Autodesk Inventor part; units mm, degrees
(part 4 of 4)
  arc A543 (17.8769, 14.9832) -> (17.4024, 14.8775) centre (19.2881, 7.5282) ccw projected
  arc A544 (17.4024, 14.8775) -> (17.024, 14.7679) centre (18.9945, 8.6707) ccw projected
  arc A545 (17.024, 14.7679) -> (16.7289, 14.6628) centre (18.6448, 9.7513) ccw projected
  arc A546 (16.7289, 14.6628) -> (16.506, 14.9696) centre (0.9435, 3.4284) ccw projected
  arc A547 (16.506, 14.9696) -> (16.6971, 15.2177) centre (12.4269, 18.3094) ccw projected
  arc A548 (16.6971, 15.2177) -> (16.9183, 15.5438) centre (11.5073, 18.976) ccw projected
  arc A549 (16.9183, 15.5438) -> (17.1654, 15.9624) centre (10.5114, 19.6082) ccw projected
  arc A550 (17.1654, 15.9624) -> (16.9181, 16.2761) centre (0.9435, 3.4284) ccw projected
  arc A551 (16.9181, 16.2761) -> (16.4534, 16.1335) centre (18.9098, 8.9549) ccw projected
  arc A552 (16.4534, 16.1335) -> (16.0847, 15.9946) centre (18.5276, 10.0708) ccw projected
  arc A553 (16.0847, 15.9946) -> (15.7988, 15.8667) centre (18.0941, 11.1207) ccw projected
  arc A554 (15.7988, 15.8667) -> (15.5525, 16.1551) centre (0.9435, 3.4284) ccw projected
  arc A555 (15.5525, 16.1551) -> (15.7236, 16.4174) centre (11.224, 19.1645) ccw projected
  arc A556 (15.7236, 16.4174) -> (15.9185, 16.7598) centre (10.2549, 19.7569) ccw projected
  arc A557 (15.9185, 16.7598) -> (16.132, 17.1965) centre (9.2125, 20.309) ccw projected
  arc A558 (16.132, 17.1965) -> (15.8608, 17.4899) centre (0.9435, 3.4284) ccw projected
  arc A559 (15.8608, 17.4899) -> (15.4087, 17.3113) centre (18.4209, 10.3475) ccw projected
  arc A560 (15.4087, 17.3113) -> (15.0521, 17.1438) centre (17.9522, 11.43) ccw projected
  arc A561 (15.0521, 17.1438) -> (14.7772, 16.9939) centre (17.4377, 12.4426) ccw projected
  arc A562 (14.7772, 16.9939) -> (14.509, 17.2621) centre (0.9435, 3.4284) ccw projected
  arc A563 (14.509, 17.2621) -> (14.6589, 17.537) centre (9.9577, 19.9226) ccw projected
  arc A564 (14.6589, 17.537) -> (14.8264, 17.8936) centre (8.9451, 20.4371) ccw projected
  arc A565 (14.8264, 17.8936) -> (15.005, 18.3458) centre (7.8625, 20.9058) ccw projected
  arc A566 (15.005, 18.3458) -> (14.7116, 18.6169) centre (0.9435, 3.4284) ccw projected
  arc A567 (14.7116, 18.6169) -> (14.2749, 18.4034) centre (17.8241, 11.6974) ccw projected
  arc A568 (14.2749, 18.4034) -> (13.9325, 18.2085) centre (17.272, 12.7398) ccw projected
  arc A569 (13.9325, 18.2085) -> (13.6702, 18.0374) centre (16.6796, 13.7089) ccw projected
  arc A570 (13.6702, 18.0374) -> (13.3818, 18.2837) centre (0.9435, 3.4284) ccw projected
  arc A571 (13.3818, 18.2837) -> (13.5097, 18.5696) centre (8.6357, 20.579) ccw projected
  arc A572 (13.5097, 18.5696) -> (13.6486, 18.9383) centre (7.5859, 21.0125) ccw projected
  arc A573 (13.6486, 18.9383) -> (13.7912, 19.403) centre (6.47, 21.3947) ccw projected
  arc A574 (13.7912, 19.403) -> (13.4775, 19.6503) centre (0.9435, 3.4284) ccw projected
  arc A575 (13.4775, 19.6503) -> (13.0589, 19.4032) centre (17.1233, 12.9963) ccw projected
  arc A576 (13.0589, 19.4032) -> (12.7328, 19.182) centre (16.4911, 13.9922) ccw projected
  arc A577 (12.7328, 19.182) -> (12.4847, 18.9909) centre (15.8245, 14.9118) ccw projected
  arc A578 (12.4847, 18.9909) -> (12.1779, 19.2138) centre (0.9435, 3.4284) ccw projected
  arc A579 (12.1779, 19.2138) -> (12.283, 19.5089) centre (7.2664, 21.1297) ccw projected
  arc A580 (12.283, 19.5089) -> (12.3926, 19.8873) centre (6.1858, 21.4794) ccw projected
  arc A581 (12.3926, 19.8873) -> (12.4983, 20.3618) centre (5.0433, 21.773) ccw projected
  arc A582 (12.4983, 20.3618) -> (12.1661, 20.5837) centre (0.9435, 3.4284) ccw projected
  arc A583 (12.1661, 20.5837) -> (11.7682, 20.3045) centre (16.3227, 14.2363) ccw projected
  arc A584 (11.7682, 20.3045) -> (11.4605, 20.0585) centre (15.6143, 15.1795) ccw projected
  arc A585 (11.4605, 20.0585) -> (11.2281, 19.8485) centre (14.8777, 16.044) ccw projected
  arc A586 (11.2281, 19.8485) -> (10.9048, 20.0466) centre (0.9435, 3.4284) ccw projected
  arc A587 (10.9048, 20.0466) -> (10.9864, 20.349) centre (5.8581, 21.5712) ccw projected
  arc A588 (10.9864, 20.349) -> (11.0659, 20.7348) centre (4.7534, 21.8351) ccw projected
  arc A589 (11.0659, 20.7348) -> (11.1341, 21.2162) centre (3.5914, 22.0381) ccw projected
  arc A590 (11.1341, 21.2162) -> (10.7855, 21.4113) centre (0.9435, 3.4284) ccw projected
  arc A591 (10.7855, 21.4113) -> (10.4107, 21.1018) centre (15.4274, 15.4096) ccw projected
  arc A592 (10.4107, 21.1018) -> (10.1233, 20.8323) centre (14.6471, 16.2943) ccw projected
  arc A593 (10.1233, 20.8323) -> (9.9081, 20.6048) centre (13.8449, 17.0984) ccw projected
  arc A594 (9.9081, 20.6048) -> (9.5702, 20.7769) centre (0.9435, 3.4284) ccw projected
  arc A595 (9.5702, 20.7769) -> (9.6279, 21.0848) centre (4.4195, 21.9009) ccw projected
  arc A596 (9.6279, 21.0848) -> (9.6769, 21.4757) centre (3.2975, 22.0773) ccw projected
  arc A597 (9.6769, 21.4757) -> (9.707, 21.9609) centre (2.1231, 22.1885) ccw projected
  arc A598 (9.707, 21.9609) -> (9.3443, 22.1281) centre (0.9435, 3.4284) ccw projected
  arc A599 (9.3443, 22.1281) -> (8.9949, 21.7901) centre (14.4427, 16.5091) ccw projected
  arc A600 (8.9949, 21.7901) -> (8.7295, 21.4989) centre (13.5955, 17.3298) ccw projected
  arc A601 (8.7295, 21.4989) -> (8.5329, 21.2552) centre (12.7326, 18.0685) ccw projected
  arc A602 (8.5329, 21.2552) -> (8.1825, 21.4003) centre (0.9435, 3.4284) ccw projected
  arc A603 (8.1825, 21.4003) -> (8.2158, 21.7117) centre (2.9594, 22.1166) ccw projected
  arc A604 (8.2158, 21.7117) -> (8.234, 22.1053) centre (1.827, 22.2045) ccw projected
  arc A605 (8.234, 22.1053) -> (8.226, 22.5913) centre (0.6476, 22.2232) ccw projected
  arc A606 (8.226, 22.5913) -> (7.8512, 22.7296) centre (0.9435, 3.4284) ccw projected
  arc A607 (7.8512, 22.7296) -> (7.5294, 22.3652) centre (13.3748, 17.5279) ccw projected
  arc A608 (7.5294, 22.3652) -> (7.2877, 22.0541) centre (12.4658, 18.2796) ccw projected
  arc A609 (7.2877, 22.0541) -> (7.1108, 21.7957) centre (11.5476, 18.9483) ccw projected
  arc A610 (7.1108, 21.7957) -> (6.7501, 21.9129) centre (0.9435, 3.4284) ccw projected
  arc A611 (6.7501, 21.9129) -> (6.7589, 22.2259) centre (1.487, 22.2172) ccw projected
  arc A612 (6.7589, 22.2259) -> (6.7462, 22.6197) centre (0.3512, 22.2159) ccw projected
  arc A613 (6.7462, 22.6197) -> (6.7, 23.1036) centre (-0.8261, 22.142) ccw projected
  arc A614 (6.7, 23.1036) -> (6.3156, 23.212) centre (0.9435, 3.4284) ccw projected
  arc A615 (6.3156, 23.212) -> (6.0234, 22.8235) centre (12.2302, 18.4597) ccw projected
  arc A616 (6.0234, 22.8235) -> (5.8068, 22.4944) centre (11.265, 19.1379) ccw projected
  arc A617 (5.8068, 22.4944) -> (5.6507, 22.2229) centre (10.2973, 19.7324) ccw projected
  arc A618 (5.6507, 22.2229) -> (5.2819, 22.3115) centre (0.9435, 3.4284) ccw projected
  arc A619 (5.2819, 22.3115) -> (5.2661, 22.6242) centre (0.0111, 22.2019) ccw projected
  arc A620 (5.2661, 22.6242) -> (5.2225, 23.0158) centre (-1.121, 22.1115) ccw projected
  arc A621 (5.2225, 23.0158) -> (5.1386, 23.4946) centre (-2.2889, 21.9455) ccw projected
  arc A622 (5.1386, 23.4946) -> (4.7468, 23.5725) centre (0.9435, 3.4284) ccw projected
  arc A623 (4.7468, 23.5725) -> (4.486, 23.1623) centre (11.0161, 19.299) ccw projected
  arc A624 (4.486, 23.1623) -> (4.2959, 22.8172) centre (10.0007, 19.8993) ccw projected
  arc A625 (4.2959, 22.8172) -> (4.1616, 22.5343) centre (8.9892, 20.4161) ccw projected
  arc A626 (4.1616, 22.5343) -> (3.787, 22.5936) centre (0.9435, 3.4284) ccw projected
  arc A627 (3.787, 22.5936) -> (3.7467, 22.9042) centre (-1.4589, 22.0709) ccw projected
  arc A628 (3.7467, 22.9042) -> (3.6725, 23.2911) centre (-2.5805, 21.8919) ccw projected
  arc A629 (3.6725, 23.2911) -> (3.5513, 23.7619) centre (-3.7318, 21.6348) ccw projected
  arc A630 (3.5513, 23.7619) -> (3.1546, 23.8088) centre (0.9435, 3.4284) ccw projected
  arc A631 (3.1546, 23.8088) -> (2.9268, 23.3794) centre (9.7398, 20.0403) ccw projected
  arc A632 (2.9268, 23.3794) -> (2.7643, 23.0205) centre (8.6805, 20.5591) ccw projected
  arc A633 (2.7643, 23.0205) -> (2.6526, 22.7279) centre (7.6316, 20.995) ccw projected
  arc A634 (2.6526, 22.7279) -> (2.2746, 22.7577) centre (0.9435, 3.4284) ccw projected
  arc A635 (2.2746, 22.7577) -> (2.21, 23.0641) centre (-2.9142, 21.8249) ccw projected
  arc A636 (2.21, 23.0641) -> (2.1057, 23.444) centre (-4.0183, 21.5585) ccw projected
  arc A637 (2.1057, 23.444) -> (1.9479, 23.9038) centre (-5.1458, 21.2118) ccw projected
  arc A638 (1.9479, 23.9038) -> (1.5487, 23.9195) centre (0.9435, 3.4284) ccw projected
  arc A639 (1.5487, 23.9195) -> (1.3553, 23.4735) centre (8.4094, 20.6793) ccw projected
  arc A640 (1.3553, 23.4735) -> (1.2215, 23.1029) centre (7.3125, 21.1133) ccw projected
  circle A641 centre (0.9435, 3.4284) radius 20.5
  circle A642 centre (0.9435, 3.4284) radius 18.25
  circle A643 centre (0.9435, 3.4284) radius 5
  point P0 (0, 0)
  dimension "d5" = 41
  dimension "d6" = 2.25
  dimension "d7" = 10
  constraints: 3 centre point, 2 coincident
  measures "d5" diameter of A641
  measures "d6" radial gap between concentric circles of A641 A642
  measures "d7" diameter of A643
extrude "押し出し3" cut sketch "スケッチ3" against normal blind 0.75 contours A0 | A642
sketch "スケッチ4" plane through (0, 0, 0) normal (0, 0, -1) x (-1, 0, 0)
  circle A0 centre (-0.9435, 3.4284) radius 8 projected
  circle A1 centre (-0.9435, 3.4284) radius 18.25
  circle A2 centre (-0.9435, 3.4284) radius 5
  point P0 (0, 0)
  dimension "d10" = 36.5
  dimension "d11" = 10
  constraints: 2 centre point, 2 coincident
  measures "d10" diameter of A1
  measures "d11" diameter of A2
extrude "押し出し4" cut sketch "スケッチ4" against normal blind 0.75 contours A0 | A1
sketch "スケッチ5" plane through (0.9435, 3.4284, 0.75) normal (0, 0, -1) x (-1, 0, 0)
  circle A0 centre (-14, 0) radius 1.25
  circle A1 centre (0, 14) radius 1.25
  circle A2 centre (14, 0) radius 1.25
  circle A3 centre (0, -14) radius 1.25
  circle A4 centre (0, 0) radius 17.5 projected
  arc A5 (-1.7867, -11.2539) -> (-1.3867, -10.4941) centre (-4.7153, -9.2268) ccw projected
  arc A6 (-1.3867, -10.4941) -> (-1.3184, -10.2522) centre (-2.5769, -10.0277) ccw projected
  line L0 (-1.3184, -10.2522) -> (-1.0841, -8.4306) projected
  arc A7 (-1.0841, -8.4306) -> (1.0841, -8.4306) centre (0, 0) ccw projected
  line L1 (1.0841, -8.4306) -> (1.3184, -10.2522) projected
  arc A8 (1.3184, -10.2522) -> (1.3867, -10.4941) centre (2.5769, -10.0277) ccw projected
  arc A9 (1.3867, -10.4941) -> (1.7867, -11.2539) centre (4.7153, -9.2268) ccw projected
  arc A10 (1.7867, -11.2539) -> (3.0777, -12.6304) centre (7.0036, -7.6547) ccw projected
  arc A11 (3.0777, -12.6304) -> (4.2394, -12.2893) centre (0, 0) ccw projected
  arc A12 (4.2394, -12.2893) -> (4.5813, -10.4334) centre (-1.7533, -10.226) ccw projected
  arc A13 (4.5813, -10.4334) -> (4.507, -9.5779) centre (1.0216, -10.3114) ccw projected
  arc A14 (4.507, -9.5779) -> (4.4336, -9.3375) centre (3.2536, -9.829) ccw projected
  line L2 (4.4336, -9.3375) -> (3.6459, -7.6784) projected
  arc A15 (3.6459, -7.6784) -> (5.47, -6.5061) centre (0, 0) ccw projected
  line L3 (5.47, -6.5061) -> (6.6519, -7.9119) projected
  arc A16 (6.6519, -7.9119) -> (6.8401, -8.0785) centre (7.5892, -7.0426) ccw projected
  arc A17 (6.8401, -8.0785) -> (7.5874, -8.5014) centre (8.9551, -5.2128) ccw projected
  arc A18 (7.5874, -8.5014) -> (9.4177, -8.9614) centre (10.0302, -2.6531) ccw projected
  arc A19 (9.4177, -8.9614) -> (10.2105, -8.0465) centre (0, 0) ccw projected
  arc A20 (10.2105, -8.0465) -> (9.4947, -6.3003) centre (4.0536, -9.5506) ccw projected
  arc A21 (9.4947, -6.3003) -> (8.9697, -5.6208) centre (6.4342, -8.1221) ccw projected
  arc A22 (8.9697, -5.6208) -> (8.778, -5.4582) centre (8.051, -6.5096) ccw projected
  line L4 (8.778, -5.4582) -> (7.2184, -4.4884) projected
  arc A23 (7.2184, -4.4884) -> (8.1191, -2.516) centre (0, 0) ccw projected
  line L5 (8.1191, -2.516) -> (9.8734, -3.0597) projected
  arc A24 (9.8734, -3.0597) -> (10.1218, -3.0981) centre (10.192, -1.8216) ccw projected
  arc A25 (10.1218, -3.0981) -> (10.9792, -3.0498) centre (10.3518, 0.4562) ccw projected
  arc A26 (10.9792, -3.0498) -> (12.7676, -2.4473) centre (9.8724, 3.1908) ccw projected
  arc A27 (12.7676, -2.4473) -> (12.9399, -1.2489) centre (0, 0) ccw projected
  arc A28 (12.9399, -1.2489) -> (11.3937, -0.1669) centre (8.5735, -5.8429) ccw projected
  arc A29 (11.3937, -0.1669) -> (10.5846, 0.1209) centre (9.8039, -3.3542) ccw projected
  arc A30 (10.5846, 0.1209) -> (10.3355, 0.1541) centre (10.2923, -1.1236) ccw projected
  line L6 (10.3355, 0.1541) -> (8.4991, 0.1267) projected
  arc A31 (8.4991, 0.1267) -> (8.1905, 2.2729) centre (0, 0) ccw projected
  line L7 (8.1905, 2.2729) -> (9.9602, 2.764) projected
  arc A32 (9.9602, 2.764) -> (10.1899, 2.866) centre (9.5589, 3.9777) ccw projected
  arc A33 (10.1899, 2.866) -> (10.8851, 3.3701) centre (8.4618, 5.9804) ccw projected
  arc A34 (10.8851, 3.3701) -> (12.0639, 4.8439) centre (6.5801, 8.0217) ccw projected
  arc A35 (12.0639, 4.8439) -> (11.5609, 5.9452) centre (0, 0) ccw projected
  arc A36 (11.5609, 5.9452) -> (9.6752, 6.0194) centre (10.3714, -0.2802) ccw projected
  arc A37 (9.6752, 6.0194) -> (8.839, 5.8242) centre (10.061, 2.4787) ccw projected
  arc A38 (8.839, 5.8242) -> (8.6115, 5.7174) centre (9.2659, 4.6193) ccw projected
  line L8 (8.6115, 5.7174) -> (7.0814, 4.7015) projected
  arc A39 (7.0814, 4.7015) -> (5.6614, 6.3402) centre (0, 0) ccw projected
  line L9 (5.6614, 6.3402) -> (6.8847, 7.7101) projected
  arc A40 (6.8847, 7.7101) -> (7.0228, 7.9201) centre (5.8909, 8.5142) ccw projected
  arc A41 (7.0228, 7.9201) -> (7.3351, 8.7201) centre (3.8853, 9.6058) ccw projected
  arc A42 (7.3351, 8.7201) -> (7.53, 10.5972) centre (1.1987, 10.3057) ccw projected
  arc A43 (7.53, 10.5972) -> (6.5115, 11.2517) centre (0, 0) ccw projected
  arc A44 (6.5115, 11.2517) -> (4.885, 10.2947) centre (8.8765, 5.3715) ccw projected
  arc A45 (4.885, 10.2947) -> (4.287, 9.6783) centre (7.1238, 7.5246) ccw projected
  arc A46 (4.287, 9.6783) -> (4.1534, 9.4655) centre (5.2976, 8.8955) ccw projected
  line L10 (4.1534, 9.4655) -> (3.4154, 7.7836) projected
  arc A47 (3.4154, 7.7836) -> (1.3349, 8.3945) centre (0, 0) ccw projected
  line L11 (1.3349, 8.3945) -> (1.6234, 10.2083) projected
  arc A48 (1.6234, 10.2083) -> (1.626, 10.4597) centre (0.3526, 10.3475) ccw projected
  arc A49 (1.626, 10.4597) -> (1.4563, 11.3015) centre (-1.9248, 10.1815) ccw projected
  arc A50 (1.4563, 11.3015) -> (0.6053, 12.9859) centre (-4.5633, 9.3178) ccw projected
  arc A51 (0.6053, 12.9859) -> (-0.6053, 12.9859) centre (0, 0) ccw projected
  arc A52 (-0.6053, 12.9859) -> (-1.4563, 11.3015) centre (4.5633, 9.3178) ccw projected
  arc A53 (-1.4563, 11.3015) -> (-1.626, 10.4597) centre (1.9248, 10.1815) ccw projected
  arc A54 (-1.626, 10.4597) -> (-1.6234, 10.2083) centre (-0.3526, 10.3475) ccw projected
  line L12 (-1.6234, 10.2083) -> (-1.3349, 8.3945) projected
  arc A55 (-1.3349, 8.3945) -> (-3.4154, 7.7836) centre (0, 0) ccw projected
  line L13 (-3.4154, 7.7836) -> (-4.1534, 9.4655) projected
  arc A56 (-4.1534, 9.4655) -> (-4.287, 9.6783) centre (-5.2976, 8.8955) ccw projected
  arc A57 (-4.287, 9.6783) -> (-4.885, 10.2947) centre (-7.1238, 7.5246) ccw projected
  arc A58 (-4.885, 10.2947) -> (-6.5115, 11.2517) centre (-8.8765, 5.3715) ccw projected
  arc A59 (-6.5115, 11.2517) -> (-7.53, 10.5972) centre (0, 0) ccw projected
  arc A60 (-7.53, 10.5972) -> (-7.3351, 8.7201) centre (-1.1987, 10.3057) ccw projected
  arc A61 (-7.3351, 8.7201) -> (-7.0228, 7.9201) centre (-3.8853, 9.6058) ccw projected
  arc A62 (-7.0228, 7.9201) -> (-6.8847, 7.7101) centre (-5.8909, 8.5142) ccw projected
  line L14 (-6.8847, 7.7101) -> (-5.6614, 6.3402) projected
  arc A63 (-5.6614, 6.3402) -> (-7.0814, 4.7015) centre (0, 0) ccw projected
  line L15 (-7.0814, 4.7015) -> (-8.6115, 5.7174) projected
  arc A64 (-8.6115, 5.7174) -> (-8.839, 5.8242) centre (-9.2659, 4.6193) ccw projected
  arc A65 (-8.839, 5.8242) -> (-9.6752, 6.0194) centre (-10.061, 2.4787) ccw projected
  arc A66 (-9.6752, 6.0194) -> (-11.5609, 5.9452) centre (-10.3714, -0.2802) ccw projected
  arc A67 (-11.5609, 5.9452) -> (-12.0639, 4.8439) centre (0, 0) ccw projected
  arc A68 (-12.0639, 4.8439) -> (-10.8851, 3.3701) centre (-6.5801, 8.0217) ccw projected
  arc A69 (-10.8851, 3.3701) -> (-10.1899, 2.866) centre (-8.4618, 5.9804) ccw projected
  arc A70 (-10.1899, 2.866) -> (-9.9602, 2.764) centre (-9.5589, 3.9777) ccw projected
  line L16 (-9.9602, 2.764) -> (-8.1905, 2.2729) projected
  arc A71 (-8.1905, 2.2729) -> (-8.4991, 0.1267) centre (0, 0) ccw projected
  line L17 (-8.4991, 0.1267) -> (-10.3355, 0.1541) projected
  arc A72 (-10.3355, 0.1541) -> (-10.5846, 0.1209) centre (-10.2923, -1.1236) ccw projected
  arc A73 (-10.5846, 0.1209) -> (-11.3937, -0.1669) centre (-9.8039, -3.3542) ccw projected
  arc A74 (-11.3937, -0.1669) -> (-12.9399, -1.2489) centre (-8.5735, -5.8429) ccw projected
  arc A75 (-12.9399, -1.2489) -> (-12.7676, -2.4473) centre (0, 0) ccw projected
  arc A76 (-12.7676, -2.4473) -> (-10.9792, -3.0498) centre (-9.8724, 3.1908) ccw projected
  arc A77 (-10.9792, -3.0498) -> (-10.1218, -3.0981) centre (-10.3518, 0.4562) ccw projected
  arc A78 (-10.1218, -3.0981) -> (-9.8734, -3.0597) centre (-10.192, -1.8216) ccw projected
  line L18 (-9.8734, -3.0597) -> (-8.1191, -2.516) projected
  arc A79 (-8.1191, -2.516) -> (-7.2184, -4.4884) centre (0, 0) ccw projected
  line L19 (-7.2184, -4.4884) -> (-8.778, -5.4582) projected
  arc A80 (-8.778, -5.4582) -> (-8.9697, -5.6208) centre (-8.051, -6.5096) ccw projected
  arc A81 (-8.9697, -5.6208) -> (-9.4947, -6.3003) centre (-6.4342, -8.1221) ccw projected
  arc A82 (-9.4947, -6.3003) -> (-10.2105, -8.0465) centre (-4.0536, -9.5506) ccw projected
  arc A83 (-10.2105, -8.0465) -> (-9.4177, -8.9614) centre (0, 0) ccw projected
  arc A84 (-9.4177, -8.9614) -> (-7.5874, -8.5014) centre (-10.0302, -2.6531) ccw projected
  arc A85 (-7.5874, -8.5014) -> (-6.8401, -8.0785) centre (-8.9551, -5.2128) ccw projected
  arc A86 (-6.8401, -8.0785) -> (-6.6519, -7.9119) centre (-7.5892, -7.0426) ccw projected
  line L20 (-6.6519, -7.9119) -> (-5.47, -6.5061) projected
  arc A87 (-5.47, -6.5061) -> (-3.6459, -7.6784) centre (0, 0) ccw projected
  line L21 (-3.6459, -7.6784) -> (-4.4336, -9.3375) projected
  arc A88 (-4.4336, -9.3375) -> (-4.507, -9.5779) centre (-3.2536, -9.829) ccw projected
  arc A89 (-4.507, -9.5779) -> (-4.5813, -10.4334) centre (-1.0216, -10.3114) ccw projected
  arc A90 (-4.5813, -10.4334) -> (-4.2394, -12.2893) centre (1.7533, -10.226) ccw projected
  arc A91 (-4.2394, -12.2893) -> (-3.0777, -12.6304) centre (0, 0) ccw projected
  arc A92 (-3.0777, -12.6304) -> (-1.7867, -11.2539) centre (-7.0036, -7.6547) ccw projected
  circle A93 centre (14, 0) radius 1.5
  circle A94 centre (0, -14) radius 1.5
  circle A95 centre (-14, 0) radius 1.5
  circle A96 centre (0, 14) radius 1.5
  line L22 (14, 0) -> (-14, 0)
  line L23 (0, 14) -> (0, -14)
  point P0 (0.9435, -3.4284)
  dimension "d14" = 3
  dimension "d15" = 3
  dimension "d16" = 3
  dimension "d17" = 3
  dimension "d27" = 28
  dimension "d28" = 28
  constraints: 8 centre point, 6 coincident, 4 end point, 2 midpoint, 1 horizontal, 1 vertical
  measures "d14" diameter of A93
  measures "d15" diameter of A94
  measures "d16" diameter of A95
  measures "d17" diameter of A96
  measures "d27" distance of L22.start L22.end
  measures "d28" distance of L23.start L23.end
extrude "押し出し5" cut sketch "スケッチ5" against normal blind 10 contours A0 | A95 | A2 | A93 | A3 | A94 | L23 A1 A50 A96 | A96 A52 A1 L23 | A96 A50 A1 A52 | L23 A51 A50 A1 | A1 A52 A51 L23 | A1 A50 A51 A52
sketch "スケッチ6" plane through (0.9435, 3.4284, 2.25) normal (0, 0, 1) x (1, 0, 0)
  circle A0 centre (14, 0) radius 1.5 projected
  circle A1 centre (-14, 0) radius 1.5 projected
  circle A2 centre (0, -14) radius 1.5 projected
  circle A3 centre (0, 14) radius 1.5 projected
  circle A4 centre (0, 0) radius 8 projected
  circle A5 centre (0, 0) radius 18.25 projected
  arc A6 (-4.4491, 13.325) -> (4.4491, 13.325) centre (0, 14) ccw
  arc A7 (13.325, 4.4491) -> (13.325, -4.4491) centre (14, 0) ccw
  arc A8 (4.4491, -13.325) -> (-4.4491, -13.325) centre (0, -14) ccw
  arc A9 (-13.325, -4.4491) -> (-13.325, 4.4491) centre (-14, 0) ccw
  arc A10 (13.325, 4.4491) -> (4.4491, 13.325) centre (0, 0) ccw
  arc A11 (4.4491, -13.325) -> (13.325, -4.4491) centre (0, 0) ccw
  arc A12 (-4.4491, 13.325) -> (-13.325, 4.4491) centre (0, 0) ccw
  arc A13 (-13.325, -4.4491) -> (-4.4491, -13.325) centre (0, 0) ccw
  point P0 (-0.9435, -3.4284)
  dimension "d20" = 3
  dimension "d21" = 3
  dimension "d22" = 3
  dimension "d23" = 3
  constraints: 16 point on circle, 8 centre point, 1 coincident
  measures "d20" radial gap between concentric circles of A3 A6
  measures "d21" radial gap between concentric circles of A0 A7
  measures "d22" radial gap between concentric circles of A2 A8
  measures "d23" radial gap between concentric circles of A1 A9
extrude "押し出し6" cut sketch "スケッチ6" against normal blind 10 contours A6 A10 A7 A11 A8 A13 A9 A12
fillet "フィレット1" radius 1 8 edges at (-3.5056, 16.7534, 1.5) (5.3926, 16.7534, 1.5) (-12.3815, 7.8775, 1.5) (-12.3815, -1.0207, 1.5) (-3.5056, -9.8966, 1.5) (5.3926, -9.8966, 1.5) (14.2685, -1.0207, 1.5) (14.2685, 7.8775, 1.5)
sketch "スケッチ7" plane through (0.9435, 3.4284, 2.25) normal (0, 0, 1) x (1, 0, 0)
  arc A0 (-5.5162, 12.9198) -> (-12.9198, 5.5162) centre (0, 0) ccw projected
  arc A1 (-4.192, 12.3637) -> (-5.5162, 12.9198) centre (-5.1235, 12.0001) ccw projected
  arc A2 (-4.192, 12.3637) -> (4.192, 12.3637) centre (0, 14) ccw projected
  arc A3 (5.5162, 12.9198) -> (4.192, 12.3637) centre (5.1235, 12.0001) ccw projected
  arc A4 (12.9198, 5.5162) -> (5.5162, 12.9198) centre (0, 0) ccw projected
  arc A5 (12.3637, 4.192) -> (12.9198, 5.5162) centre (12.0001, 5.1235) ccw projected
  arc A6 (12.3637, 4.192) -> (12.3637, -4.192) centre (14, 0) ccw projected
  arc A7 (12.9198, -5.5162) -> (12.3637, -4.192) centre (12.0001, -5.1235) ccw projected
  arc A8 (5.5162, -12.9198) -> (12.9198, -5.5162) centre (0, 0) ccw projected
  arc A9 (4.192, -12.3637) -> (5.5162, -12.9198) centre (5.1235, -12.0001) ccw projected
  arc A10 (4.192, -12.3637) -> (-4.192, -12.3637) centre (0, -14) ccw projected
  arc A11 (-5.5162, -12.9198) -> (-4.192, -12.3637) centre (-5.1235, -12.0001) ccw projected
  arc A12 (-12.9198, -5.5162) -> (-5.5162, -12.9198) centre (0, 0) ccw projected
  arc A13 (-12.3637, -4.192) -> (-12.9198, -5.5162) centre (-12.0001, -5.1235) ccw projected
  arc A14 (-12.3637, -4.192) -> (-12.3637, 4.192) centre (-14, 0) ccw projected
  arc A15 (-12.9198, 5.5162) -> (-12.3637, 4.192) centre (-12.0001, 5.1235) ccw projected
  circle A16 centre (14, 0) radius 1.5 projected
  circle A17 centre (-14, 0) radius 1.5 projected
  circle A18 centre (0, -14) radius 1.5 projected
  circle A19 centre (0, 14) radius 1.5 projected
  circle A20 centre (0, 0) radius 18.25 projected
